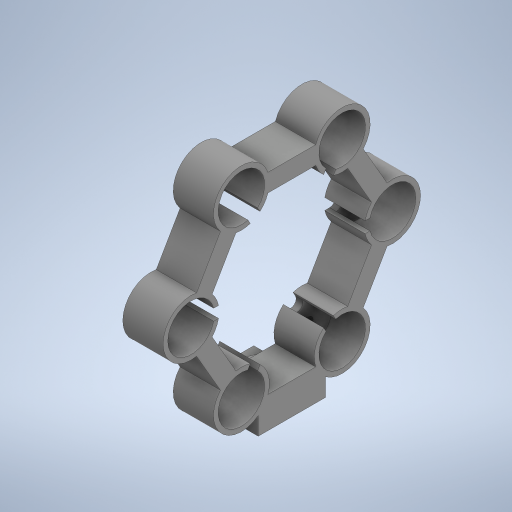
# Autodesk Inventor part: support_electrical_magnets
Saved by Autodesk Inventor 2023 (Build 270158000, 158)
## iProperties
Created: 2022-11-02
Part Number: support_electrical_magnets
Material: Generic
Document SubType Name: Modeling
Designer: Admin
Density: 1 g/cm^3
Appearance: Default
Author: Admin
Autodesk Inventor part; units mm, degrees
ref_plane "YZ Plane" through (0, 0, 0) normal (1, 0, 0) x (0, 1, 0)
ref_plane "XZ Plane" through (0, 0, 0) normal (0, 1, 0) x (-1, 0, 0)
ref_plane "XY Plane" through (0, 0, 0) normal (0, 0, 1) x (1, 0, 0)
sketch "Sketch1" plane through (0, 0, 0) normal (1, 0, 0) x (0, 1, 0)
  line L0 (38.9711, 22.5) -> (38.9711, -22.5)
  line L1 (38.9711, -22.5) -> (0, -45)
  line L2 (0, -45) -> (-38.9711, -22.5)
  line L3 (-38.9711, -22.5) -> (-38.9711, 22.5)
  line L4 (-38.9711, 22.5) -> (0, 45)
  line L5 (0, 45) -> (38.9711, 22.5)
  line L6 (0, 45) -> (0, -45)
  line L7 (38.9711, 0) -> (-38.9711, 0)
  circle A0 centre (38.9711, -22.5) radius 17.5
  circle A1 centre (38.9711, -22.5) radius 12.5
  circle A2 centre (38.9711, -22.5) radius 10.4
  circle A3 centre (38.9711, -22.5) radius 15
  line L8 (38.9711, -22.5) -> (62.5188, -22.5)
  line L9 (53.9711, -26.5) -> (61.9711, -26.5)
  line L10 (61.9711, -26.5) -> (61.9711, -18.5)
  line L11 (61.9711, -18.5) -> (53.9711, -18.5)
  line L12 (53.9711, -18.5) -> (53.9711, -26.5)
  line L13 (53.9711, -26.5) -> (61.9711, -18.5) construction
  line L14 (61.9711, -26.5) -> (53.9711, -18.5) construction
  circle A4 centre (38.9711, 22.5) radius 10.4
  circle A5 centre (38.9711, 22.5) radius 12.5
  circle A6 centre (0, 45) radius 10.4
  circle A7 centre (0, 45) radius 12.5
  circle A8 centre (-38.9711, 22.5) radius 10.4
  circle A9 centre (-38.9711, 22.5) radius 12.5
  circle A10 centre (-38.9711, -22.5) radius 10.4
  circle A11 centre (-38.9711, -22.5) radius 12.5
  circle A12 centre (0, -45) radius 10.4
  circle A13 centre (0, -45) radius 12.5
  line L15 (42.9711, 10.6573) -> (42.9711, -10.6573)
  line L16 (34.9711, 10.6573) -> (34.9711, -10.6573)
  line L17 (12.2561, 42.5427) -> (30.715, 31.8855)
  line L18 (8.2561, 35.6145) -> (26.715, 24.9573)
  line L19 (-30.715, 31.8855) -> (-12.2561, 42.5427)
  line L20 (-26.715, 24.9573) -> (-8.2561, 35.6145)
  line L21 (-42.9711, -10.6573) -> (-42.9711, 10.6573)
  line L22 (-34.9711, -10.6573) -> (-34.9711, 10.6573)
  line L23 (-12.2561, -42.5427) -> (-30.715, -31.8855)
  line L24 (-8.2561, -35.6145) -> (-26.715, -24.9573)
  line L25 (30.715, -31.8855) -> (12.2561, -42.5427)
  line L26 (26.715, -24.9573) -> (8.2561, -35.6145)
  line L27 (38.9711, 22.5) -> (0, 0)
  line L28 (28.9786, 19.6175) -> (27.1145, 18.5413)
  line L29 (31.4786, 15.2874) -> (29.6145, 14.2112)
  line L30 (29.9645, 17.3) -> (28.1458, 16.25)
  arc A14 (31.4786, 15.2874) -> (28.9786, 19.6175) centre (30.2286, 17.4525) ccw
  arc A15 (27.1145, 18.5413) -> (29.6145, 14.2112) centre (28.3645, 16.3763) ccw
  arc A16 (2.5, 34.905) -> (-2.5, 34.905) centre (0, 34.905) ccw
  line L31 (2.5, 34.905) -> (2.5, 32.7526)
  line L32 (-2.5, 34.905) -> (-2.5, 32.7526)
  arc A17 (-2.5, 32.7526) -> (2.5, 32.7526) centre (0, 32.7526) ccw
  arc A18 (-28.9786, 19.6175) -> (-31.4786, 15.2874) centre (-30.2286, 17.4525) ccw
  line L33 (-28.9786, 19.6175) -> (-27.1145, 18.5413)
  line L34 (-31.4786, 15.2874) -> (-29.6145, 14.2112)
  arc A19 (-29.6145, 14.2112) -> (-27.1145, 18.5413) centre (-28.3645, 16.3763) ccw
  arc A20 (-31.4786, -15.2874) -> (-28.9786, -19.6175) centre (-30.2286, -17.4525) ccw
  line L35 (-31.4786, -15.2874) -> (-29.6145, -14.2112)
  line L36 (-28.9786, -19.6175) -> (-27.1145, -18.5413)
  arc A21 (-27.1145, -18.5413) -> (-29.6145, -14.2112) centre (-28.3645, -16.3763) ccw
  arc A22 (-2.5, -34.905) -> (2.5, -34.905) centre (0, -34.905) ccw
  line L37 (-2.5, -34.905) -> (-2.5, -32.7526)
  line L38 (2.5, -34.905) -> (2.5, -32.7526)
  arc A23 (2.5, -32.7526) -> (-2.5, -32.7526) centre (0, -32.7526) ccw
  arc A24 (28.9786, -19.6175) -> (31.4786, -15.2874) centre (30.2286, -17.4525) ccw
  line L39 (28.9786, -19.6175) -> (27.1145, -18.5413)
  line L40 (31.4786, -15.2874) -> (29.6145, -14.2112)
  arc A25 (29.6145, -14.2112) -> (27.1145, -18.5413) centre (28.3645, -16.3763) ccw
  line L41 (-48.9711, -15) -> (-48.9711, 15)
  line L42 (-48.9711, 15) -> (-56.9711, 15)
  line L43 (-56.9711, 15) -> (-56.9711, -15)
  line L44 (-56.9711, -15) -> (-48.9711, -15)
  circle A26 centre (-38.9711, -22.5) radius 17.5
  circle A27 centre (-38.9711, 22.5) radius 17.5
  line L45 (-52.9711, -15) -> (-52.9711, 15)
  circle A28 centre (38.9711, 22.5) radius 2
  circle A29 centre (0, 45) radius 2
  circle A30 centre (-38.9711, 22.5) radius 2
  circle A31 centre (-38.9711, -22.5) radius 2
  circle A32 centre (0, -45) radius 2
  circle A33 centre (38.9711, -22.5) radius 2
  point P0 (57.9711, -22.5)
  point P1 (-42.9711, 10.6573)
  dimension "d0" = 35
  dimension "d1" = 45
  dimension "d2" = 25
  dimension "d3" = 20.8
  dimension "d4" = 30
  dimension "d5" = 8
  dimension "d6" = 8
  dimension "d9" = 360
  dimension "d11" = 4
  dimension "d12" = 4
  dimension "d15" = 360
  dimension "d17" = 2.5
  dimension "d18" = 2.5
  dimension "d22" = 360
  dimension "d24" = 30
  dimension "d25" = 8
  dimension "d26" = 30
  dimension "d28" = 35
  dimension "d29" = 35
  dimension "d30" = 4
  dimension "d35" = 4
  dimension "d38" = 360
  constraints: 92 end point, 36 point on circle, 33 centre point, 13 coincident, 6 midpoint, 4 parallel, 3 horizontal, 3 perpendicular, 3 point on line, 3 tangent, 3 vertical, 152 other
  measures "d0" diameter of A0
  measures "d1" distance of L0.start L0.end
  measures "d2" diameter of A1
  measures "d3" diameter of A2
  measures "d4" diameter of A3
  measures "d5" distance of L11.end L10.end
  measures "d6" distance of L9.end L10.end
  measures "d11" distance between parallel lines of L15 L0
  measures "d12" distance between parallel lines of L0 L16
  measures "d17" distance between parallel lines of L27 L28
  measures "d18" distance between parallel lines of L27 L29
  measures "d24" distance of L41.start L41.end
  measures "d25" distance of L42.start L42.end
  measures "d26" distance of L42.end L43.end
  measures "d28" diameter of A26
  measures "d29" diameter of A27
  measures "d30" distance between parallel lines of L43 L45
  measures "d35" diameter of A28
extrude "Extrusion1" add sketch "Sketch1" against normal blind 18 contours L5 A28 L0 | L27 A28 L5 | L0 A28 L27 | A28 L5 A4 L0 | L0 A4 A14 L27 A28 | A28 L27 A14 A4 L5 | A4 L5 A5 L0 | L0 A5 L29 A4 | A4 L28 A5 L5 | A14 A4 L27 | L27 A4 A14 | A5 L15 A0 L0 | L0 L7 L16 A5 | L29 A5 L27 A4 | A5 L18 A7 L5 | L5 A7 L17 A5 | A4 L27 A5 L28 | L0 A0 L16 L7 | A7 L31 A6 L5 | L5 A6 L4 A7 | A0 L15 A3 L0 | L0 A3 L16 A0 | A6 A16 L6 A29 L5 | L5 A29 L4 A6 | A3 L15 A1 L0 | L0 A1 L16 A3 | A29 L6 L5 | L5 L4 A29 | L31 A7 L6 A6 | A6 L6 A16 | A1 L8 A2 L0 | L0 A2 L40 A1 | L26 A3 L1 A0 | A0 L1 A13 L26 | L6 A29 L4 | L6 A16 A6 L4 A29 | A6 A16 L6 | L6 A7 L32 A6 | A6 L32 A7 L4 | A7 L4 A27 L19 | A2 L8 A33 L0 | L0 A33 L1 A2 A24 | L26 A1 L1 A3 | A0 L25 A13 L1 | L1 A3 L25 A0 | A13 L1 A12 L38 | A13 L38 A12 L6 | L6 A12 L37 A13 | L37 A12 L2 A13 | A3 L1 A1 L25 | A1 L1 A2 L8 | A7 L20 A27 L4 | A27 L4 A9 L19 | A33 L8 L0 | L0 L1 A33 | A2 L1 A33 L8 | A24 A2 | A2 L39 A1 L40 | A1 L39 A2 L1 | A13 L2 A12 L1 | A12 A22 L6 | L6 A22 A12 | A12 L1 A32 L6 A22 | A13 L2 A26 L24 | A22 L6 A32 L2 A12 | A11 L35 A10 L3 | A9 L3 A8 L34 | A27 L20 A9 L4 | A9 L4 A8 L3 | A27 L45 A26 L44 L43 L42 | L42 L45 A27 | L8 A33 L1 | A12 L2 A32 L1 | A13 L23 A26 L2 | A26 L2 A11 L24 | L3 A10 L2 A11 | A26 L41 A27 L21 | L21 A11 L41 A26 | A27 L41 A9 L21 | A11 L36 A10 L35 | L34 A8 L33 A9 | A9 L33 A8 L4 | L41 A27 L45 L42 | A27 L41 A26 L45 | A32 L2 L1 | L1 L6 A32 | L6 L2 A32 | A26 L23 A11 L2 | A11 L2 A10 L36 | A10 A20 L2 A31 L3 | L3 A31 L2 A10 | L41 L44 L45 A26 | A8 L4 A30 L3 | L3 A30 L4 A8 A18 | A10 A20 | A18 A8 | L45 L44 A26 | A31 L2 L3 | L3 L2 A31 | A30 L4 L3 | L3 L4 A30
extrude "Extrusion2" cut sketch "Sketch1" against normal blind 15 contours L5 A28 L0 | L27 A28 L5 | L0 A28 L27 | A28 L5 A4 L0 | L0 A4 A14 L27 A28 | A28 L27 A14 A4 L5 | A14 A4 L27 | L27 A4 A14 | A6 A16 L6 A29 L5 | L5 A29 L4 A6 | A29 L6 L5 | L5 L4 A29 | A6 L6 A16 | L6 A29 L4 | L6 A16 A6 L4 A29 | A6 A16 L6 | A2 L8 A33 L0 | L0 A33 L1 A2 A24 | A33 L8 L0 | L0 L1 A33 | A2 L1 A33 L8 | A24 A2 | A12 A22 L6 | L6 A22 A12 | A12 L1 A32 L6 A22 | A22 L6 A32 L2 A12 | L8 A33 L1 | A12 L2 A32 L1 | A32 L2 L1 | L1 L6 A32 | L6 L2 A32 | A10 A20 L2 A31 L3 | L3 A31 L2 A10 | A8 L4 A30 L3 | L3 A30 L4 A8 A18 | A10 A20 | A18 A8 | A31 L2 L3 | L3 L2 A31 | A30 L4 L3 | L3 L4 A30
extrude "Extrusion3" cut sketch "Sketch1" against normal blind 18 contours L5 A28 L0 | L27 A28 L5 | L0 A28 L27 | A14 A4 L27 | L27 A4 A14 | L29 A5 L27 A4 | A4 L27 A5 L28 | A29 L6 L5 | L5 L4 A29 | L31 A7 L6 A6 | A6 L6 A16 | L6 A29 L4 | A6 A16 L6 | L6 A7 L32 A6 | A13 L38 A12 L6 | L6 A12 L37 A13 | A33 L8 L0 | L0 L1 A33 | A24 A2 | A2 L39 A1 L40 | A12 A22 L6 | L6 A22 A12 | L8 A33 L1 | A11 L36 A10 L35 | L34 A8 L33 A9 | A32 L2 L1 | L1 L6 A32 | L6 L2 A32 | A10 A20 | A18 A8 | A31 L2 L3 | L3 L2 A31 | A30 L4 L3 | L3 L4 A30
extrude "Extrusion4" add sketch "Sketch1" against normal blind 32 contours A27 L45 A26 L44 L43 L42 | L42 L45 A27 | L45 L44 A26
sketch "Sketch2" plane through (0, 0, 0) normal (0, 0, 1) x (1, 0, 0)
  line L0 (-18, -42.9711) -> (-32, -52.9711)
  line L1 (-18, -30.715) -> (-18, -51.4711) projected
  line L2 (-18, -46.6579) -> (-26.8386, -52.9711)
  line L3 (-18, -52.9711) -> (-32, -52.9711) projected
  point P0 (0, 0)
  point P1 (-18, -48.9711)
  point P2 (-22.4193, -49.8145)
  dimension "d44" = 3
  constraints: 4 end point, 2 point on line, 1 midpoint, 1 parallel
  measures "d44" distance from line of L0 point (-22.419, -49.814)
extrude "Extrusion5" add sketch "Sketch2" along normal mid plane 5
sketch "Sketch3" plane through (0, -56.9711, -15) normal (0, -1, 0) x (1, 0, 0)
  line L0 (0, 30) -> (0, 0) projected
  line L1 (0, 30) -> (-32, 30) projected
  line L2 (-32, 0) -> (-32, 30) projected
  line L3 (0, 0) -> (-32, 0) projected
  line L4 (-32, 0) -> (0, 30)
  line L5 (-6, 25) -> (-26, 25)
  line L6 (-26, 25) -> (-26, 5)
  line L7 (-26, 5) -> (-6, 5)
  line L8 (-6, 5) -> (-6, 25)
  line L9 (-6, 25) -> (-26, 5) construction
  line L10 (-26, 25) -> (-6, 5) construction
  circle A0 centre (-26, 25) radius 1.5
  circle A1 centre (-26, 5) radius 1.5
  circle A2 centre (-6, 5) radius 1.5
  circle A3 centre (-6, 25) radius 1.5
  point P0 (0, 15)
  point P1 (-16, 15)
  dimension "d47" = 20
  dimension "d48" = 20
  dimension "d49" = 3
  dimension "d52" = 360
  constraints: 14 end point, 4 centre point, 3 midpoint, 2 parallel, 1 coincident, 1 horizontal, 1 perpendicular, 9 other
  measures "d47" distance of L7.end L6.end
  measures "d48" distance of L5.end L6.end
  measures "d49" diameter of A0
extrude "Extrusion6" cut sketch "Sketch3" against normal blind 5 contours A1 L6 L4 | L4 L6 L7 A1 | A0 L6 L5 | L5 L6 A0 | L6 A1 L4 | L4 A1 L7 L6
equation "\"d6\" = d5"
equation "\"d12\" = d11"
equation "\"d18\" = d17"
body "Solid1"
